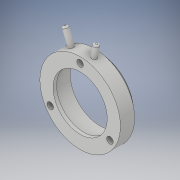
# Autodesk Inventor part: Part3
Saved by Autodesk Inventor 2017 (Build 210142000, 142)
## iProperties
Created: 2017-04-21
Part Number: Part3
Material: Generic
Document SubType Name: Modeling
Designer: 167942
Density: 1 g/cm^3
Appearance: Default
Author: 167942
Autodesk Inventor part; units mm, degrees
sketch "Sketch1" plane through (0, 0, 0) normal (1, 0, 0) x (0, 1, 0)
  line L0 (9.6583, 12.5432) -> (9.6583, -1.1759)
  line L1 (9.6583, -1.1759) -> (4.0957, -1.1759)
  line L2 (4.0957, -1.1759) -> (4.0957, -6.5068)
  line L3 (4.0957, -6.5068) -> (-0.6541, -6.5068)
  line L4 (-0.6541, -6.5068) -> (-0.6541, 9.1142)
  line L5 (-0.6541, 9.1142) -> (-3.0417, 9.1142)
  line L6 (-3.0417, 9.1142) -> (-3.0417, 12.5432)
  line L7 (-3.0417, 12.5432) -> (9.6583, 12.5432)
  line L8 (9.6583, 12.5432) -> (-29.2355, 12.5432) construction
  line L9 (-29.2355, 12.5432) -> (-29.2355, -33.1187) construction
  point P0 (0, 0)
  dimension "d0" = 12.7
  dimension "d1" = 19.05
  dimension "d2" = 5.5626
  dimension "d3" = 10.3124
  dimension "d4" = 3.429
  dimension "d5" = 38.8937
  constraints: 20 end point, 8 perpendicular, 1 horizontal, 1 vertical
  measures "d0" distance between parallel lines of L6 L0
  measures "d1" distance between parallel lines of L3 L7
  measures "d2" distance of L0.end L1.end
  measures "d3" distance between parallel lines of L4 L0
  measures "d4" distance of L5.end L6.end
  measures "d5" distance of L0.start L8.end
revolve "Revolution1" add sketch "Sketch1" angle 360 about axis through (0, -29.2355, 12.5432) along (0, 0, -1)
chamfer "Chamfer1" distance 0.7874 angle 45 1 edges at (0, -62.5666, -6.5068)
sketch "Sketch2" plane through (0, -29.2355, 12.5432) normal (0, 0, 1) x (1, 0, 0)
  circle A0 centre (0, 0) radius 38.8938 projected
  circle A1 centre (0, 0) radius 33.3312 projected
  circle A2 centre (0, 33.3312) radius 3.175
  circle A3 centre (-28.8656, -16.6656) radius 3.175
  circle A4 centre (28.8656, -16.6656) radius 3.175
  point P0 (0, 29.2355)
  dimension "d10" = 6.35
  dimension "d13" = 360
  constraints: 3 centre point, 7 other
  measures "d10" diameter of A2
extrude "Extrusion1" cut sketch "Sketch2" against normal blind 10.3124 contours A2 A1 | A1 A2 | A4 A1 | A1 A4 | A3 A1 | A1 A3
ref_plane "Work Plane1" through (0, -29.2355, 5.6836) normal (0, 0, 1) x (1, 0, 0)
sketch "Sketch4" plane through (0, -29.2355, 5.6836) normal (0, 0, 1) x (1, 0, 0)
  line L0 (0, 0) -> (0, 62.7832) construction
  circle A0 centre (0, 0) radius 28.5814 projected
  line L1 (-11.1676, 26.3093) -> (-21.5633, 50.8)
  line L2 (4.9631, 28.1471) -> (8.9574, 50.8)
  point P0 (0, 29.2355)
  dimension "d21" = 23
  dimension "d22" = 10
  dimension "d23" = 50.8
  dimension "d24" = 50.8
  constraints: 6 end point, 2 point on circle, 1 vertical
  measures "d21" angle of L0 L1
  measures "d22" angle of L0 L2
  measures "d23" vertical distance of A0.centre L1.end
  measures "d24" vertical distance of A0.centre L2.end
ref_plane "Work Plane2" through (8.9574, 21.5645, 5.6836) normal (0.1736, 0.9848, 0) x (-0.9848, 0.1736, 0)
sketch "Sketch5" plane through (8.9574, 21.5645, 5.6836) normal (0.1736, 0.9848, 0) x (-0.9848, 0.1736, 0)
  circle A0 centre (0, 0) radius 2.54
  point P0 (5.0767, -5.6836)
  dimension "d25" = 5.08
  constraints: 1 centre point
  measures "d25" diameter of A0
extrude "Extrusion2" add sketch "Sketch5" against normal blind 20.6375
ref_plane "Work Plane3" through (-21.5633, 21.5645, 5.6836) normal (-0.3907, 0.9205, 0) x (-0.9205, -0.3907, 0)
sketch "Sketch7" plane through (-21.5633, 21.5645, 5.6836) normal (-0.3907, 0.9205, 0) x (-0.9205, -0.3907, 0)
  circle A0 centre (0, 0) radius 2.54
  point P0 (-11.4232, -5.6836)
  dimension "d28" = 5.08
  constraints: 1 centre point
  measures "d28" diameter of A0
extrude "Extrusion3" add sketch "Sketch7" against normal blind 20.6375
fillet "Fillet1" radius 1.5875 1 edges at (11.4588, 21.1235, 5.6836)
fillet "Fillet2" radius 1.5875 1 edges at (-19.2252, 22.557, 5.6836)
body "Solid1"
